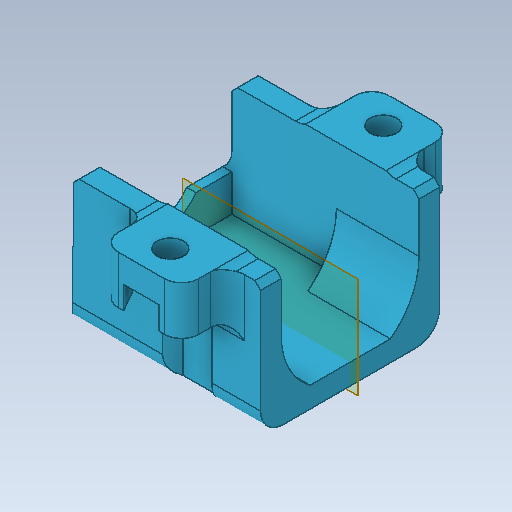
# Autodesk Inventor part: MotorTop
Saved by Autodesk Inventor 2025 (Build 290162000, 162)
## iProperties
Created: 2015-06-14
Part Number: MotorTop
Material: PC/ABS Plastic
Document SubType Name: Modeling
Designer: Lincoln
Density: 0.357273 g/cm^3
Appearance: Turquoise
Mass: 0.194626 g
Surface Area: 10.2421 cm^2
Volume: 0.544755 cm^3
Author: Lincoln
Autodesk Inventor part; units mm, degrees
ref_plane "YZ Plane" through (0, 0, 0) normal (1, 0, 0) x (0, 1, 0)
ref_plane "XZ Plane" through (0, 0, 0) normal (0, 1, 0) x (-1, 0, 0)
ref_plane "XY Plane" through (0, 0, 0) normal (0, 0, 1) x (1, 0, 0)
sketch "Sketch1" plane through (0, 0, 0) normal (1, 0, 0) x (0, 1, 0)
  line L0 (4.975, -6) -> (0, -6) construction
  line L1 (0, -6) -> (0, 0) construction
  line L2 (0, 0) -> (8.45, 0) construction
  line L3 (4.975, 6) -> (0, 6) construction
  line L4 (0, 6) -> (0, 0) construction
  line L5 (0, 6) -> (0, 7.8) construction
  line L6 (0, 7.8) -> (9.8, 7.8)
  line L7 (9.8, 7.8) -> (9.8, 6)
  line L8 (9.8, 6) -> (4.975, 6)
  line L9 (9.8, -6) -> (9.8, -7.8)
  line L10 (9.8, -7.8) -> (0, -7.8)
  line L11 (0, -7.8) -> (0, -6) construction
  line L12 (9.8, -6) -> (4.975, -6)
  line L13 (0, 7.8) -> (-1.8, 7.8)
  line L14 (-1.8, 7.8) -> (-1.8, -7.8)
  line L15 (-1.8, -7.8) -> (0, -7.8)
  circle A0 centre (4.975, -0.2001) radius 2.5 projected
  line L16 (9.95, -3.5) -> (9.95, 3.5) projected
  arc A1 (9.95, 3.5) -> (0, 3.5) centre (4.975, -0.2001) ccw projected
  line L17 (0, 3.5) -> (0, -3.5) projected
  arc A2 (0, -3.5) -> (9.95, -3.5) centre (4.975, 0.2001) ccw projected
  point P0 (0, 0)
  point P1 (4.975, 6)
  dimension "d8" = 0
  dimension "d22" = 1.8
  dimension "d23" = 9.8
  dimension "d24" = 1.8
  dimension "d25" = 1.8
  constraints: 32 end point, 7 perpendicular, 4 horizontal, 3 vertical, 1 collinear, 1 point on circle, 1 tangent, 4 other
  measures "d8" distance of L1.end point (0, 0)
  measures "d22" distance of L3.end L5.end
  measures "d23" distance of L5.end L6.end
  measures "d24" distance of L6.end L7.end
  measures "d25" distance of L5.end L13.end
extrude "Extrusion1" add sketch "Sketch1" along normal blind 15.2 contours L6 L7 L8 A1 L17 A2 L12 L9 L10 L15 L14 L13
sketch "Sketch2" plane through (0, -1.8, -7.8) normal (0, -1, 0) x (1, 0, 0)
  line L0 (-9.1, 0) -> (-9.1, 10.8)
  line L1 (-9.1, 10.8) -> (-9.1, 15.6)
  line L2 (-9.1, 15.6) -> (-9.9, 15.6)
  line L3 (-9.9, 15.6) -> (-9.9, 0)
  line L4 (-9.9, 0) -> (-9.1, 0)
  line L5 (0, 15.6) -> (15.2, 15.6) projected
  line L6 (0, 0) -> (15.2, 0) projected
  line L7 (0, 15.6) -> (0, 0) projected
  dimension "d30" = 0.8
  dimension "d141" = 9.1
  constraints: 10 end point, 3 perpendicular, 2 collinear, 1 point on line
  measures "d30" distance of L1.end L2.end
  measures "d141" distance between parallel lines of L7 L0
extrude "Extrusion2" add sketch "Sketch2" against normal blind 5
sketch "Sketch3" plane through (-9.1, -1.8, 7.8) normal (1, 0, 0) x (0, 0, -1)
  line L0 (0, 11.6) -> (0, 0) projected
  line L1 (0, 0) -> (15.6, 0) projected
  circle A0 centre (8.0001, 6.775) radius 2 projected
  arc A1 (13.8, 11.25) -> (13.3, 11.75) centre (13.3, 11.25) ccw projected
  line L2 (13.8, 11.25) -> (13.8, 2.3) projected
  arc A2 (13.3, 1.8) -> (13.8, 2.3) centre (13.3, 2.3) ccw projected
  line L3 (13.3, 1.8) -> (2.3, 1.8) projected
  arc A3 (1.8, 2.3) -> (2.3, 1.8) centre (2.3, 2.3) ccw projected
  line L4 (1.8, 2.3) -> (1.8, 11.25) projected
  arc A4 (2.3, 11.75) -> (1.8, 11.25) centre (2.3, 11.25) ccw projected
  line L5 (2.3, 11.75) -> (13.3, 11.75) projected
  line L6 (0, 11.6) -> (0, 0) projected
  line L7 (1.8, 11.6) -> (0, 11.6) projected
  line L8 (1.8, 6.775) -> (1.8, 11.6) projected
  arc A5 (1.8, 6.775) -> (4.3, 1.8) centre (8.0001, 6.775) ccw projected
  line L9 (11.3, 1.8) -> (4.3, 1.8) projected
  arc A6 (11.3, 1.8) -> (13.8, 6.775) centre (7.5999, 6.775) ccw projected
  line L10 (13.8, 11.6) -> (13.8, 6.775) projected
  line L11 (15.6, 11.6) -> (13.8, 11.6) projected
  line L12 (15.6, 0) -> (15.6, 11.6) projected
  line L13 (0, 0) -> (15.6, 0) projected
  point P0 (7.8, 1.8)
  point P1 (1.8, 9.8)
  point P2 (13.8, 9.8)
  point P3 (0, 1)
  point P4 (4.3, 1.8)
  point P5 (13.8, 6.775)
  point P6 (11.3, 1.8)
  point P7 (1.8, 6.775)
extrude "Extrusion3" add sketch "Sketch3" along normal blind 9.5 contours L7 L8 L4 A3 L3 A2 L2 L10 L11 L12 L1 L0 | A5 L3 A3 L4 | A6 L2 A2 L3
sketch "Sketch4" plane through (0, 0, 0) normal (-1, 0, 0) x (0, 0, 1)
  line L0 (-7.8, -1.8) -> (-7.8, 9.8) projected
  line L1 (-7.8, -1.8) -> (-7.8, 3.2) projected
  line L2 (-7.8, 3.2) -> (-7.8, 9.8) projected
  line L3 (7.8, 9.8) -> (7.8, -1.8) projected
  line L4 (7.8, 9.8) -> (7.8, 3.2) projected
  line L5 (7.8, -1.8) -> (7.8, 3.2) projected
  line L6 (7.8, -1.8) -> (-7.8, -1.8) projected
  line L7 (7.8, -1.8) -> (-7.8, -1.8) projected
  line L8 (-6, 9.8) -> (-6, 4.975) projected
  line L9 (-6, 9.8) -> (-6, 4.975) projected
  line L10 (6, 4.975) -> (6, 9.8) projected
  line L11 (6, 4.975) -> (6, 9.8) projected
  line L12 (-3.5, 0) -> (3.5, 0) projected
  line L13 (3.5, 0) -> (-3.5, 0) projected
  line L14 (-6, 4.975) -> (-6, 0)
  line L15 (-6, 0) -> (-3.5, 0)
  line L16 (6, 4.975) -> (6, 0)
  arc A0 (3.5, 0) -> (5.7405, 3.2) centre (-0.2001, 4.975) ccw projected
  line L17 (6, 0) -> (3.5, 0)
  line L18 (-7.8, 9.8) -> (-6, 9.8) projected
  line L19 (-7.8, 9.8) -> (-6, 9.8) projected
  line L20 (6, 9.8) -> (7.8, 9.8) projected
  line L21 (6, 9.8) -> (7.8, 9.8) projected
  arc A1 (-6, 4.975) -> (-3.5, 0) centre (0.2001, 4.975) ccw projected
  arc A2 (-6, 4.975) -> (-5.7405, 3.2) centre (0.2001, 4.975) ccw projected
  arc A3 (-5.7405, 3.2) -> (-3.5, 0) centre (0.2001, 4.975) ccw projected
  arc A4 (3.5, 0) -> (6, 4.975) centre (-0.2001, 4.975) ccw projected
  arc A5 (3.5, 0) -> (5.7405, 3.2) centre (-0.2001, 4.975) ccw projected
  arc A6 (5.7405, 3.2) -> (6, 4.975) centre (-0.2001, 4.975) ccw projected
  point P0 (0, 0)
  point P1 (-3.5, 0)
  point P2 (-6, 4.975)
  point P3 (-7.8, -1.8)
  point P4 (7.8, -1.8)
  point P5 (-3.5, 0)
  point P6 (-6, 4.975)
  constraints: 8 end point, 2 point on line, 1 horizontal, 1 perpendicular, 1 vertical
extrude "Extrusion4" cut sketch "Sketch4" along normal blind 9.1 contours A1 L15 L14 | L16 L17 A0 A4
sketch "Sketch5" plane through (15.2, 9.8, -7.8) normal (0, 0, -1) x (-1, 0, 0)
  line L0 (15.2, 0) -> (11.2, 0) construction
  line L1 (24.3, 0) -> (0, 0) construction
  line L2 (0, -11.6) -> (0, 0)
  line L3 (0, 0) -> (0, 0)
  line L4 (0, 0) -> (0, -6)
  line L5 (0, 0) -> (11.2, 0)
  line L6 (8, -11.6) -> (0, -11.6)
  line L7 (0, -11.6) -> (0, 0)
  line L8 (0, 0) -> (8, 0)
  line L9 (8, 0) -> (8, -11.6)
  line L10 (25.1, -11.6) -> (0, -11.6) projected
  dimension "d48" = 0
  dimension "d113" = 8
  constraints: 18 end point, 2 collinear, 2 parallel, 2 point on line, 1 horizontal, 1 perpendicular
  measures "d48" distance of L1.end L3.end
  measures "d113" distance between parallel lines of L2 L9
extrude "Extrusion5" cut sketch "Sketch5" against normal through all
sketch "Sketch10" plane through (0, 9.8, 7.2) normal (0, 1, 0) x (1, 0, 0)
  line L0 (-2.6843, -4.6) -> (4.3157, -4.6)
  line L1 (4.3157, -4.6) -> (4.3157, 0)
  line L2 (4.3157, 0) -> (-2.6843, 0) construction
  line L3 (-2.6843, 1.2) -> (-2.6843, -4.6)
  line L4 (0.8157, -4.6) -> (0.8157, 0) construction
  line L5 (-6.65, -2.0756) -> (1.3238, -2.0756) construction
  circle A0 centre (0.8157, -2.0756) radius 1.15
  line L6 (-5.9343, -1) -> (-5.9343, 11.4) construction
  line L7 (0, 1.2) -> (-2.6843, 1.2)
  line L8 (-9.1, 1.2) -> (7.2, 1.2) projected
  line L9 (-9.1, -0.6) -> (15.2, -0.6) projected
  circle A1 centre (0.8157, -2.0756) radius 1.1 projected
  line L10 (4.3157, 0) -> (4.3157, 1.2)
  line L11 (0, 1.2) -> (4.3157, 1.2)
  point P0 (0, 6.2)
  point P1 (0, -0.6)
  point P2 (7.2, -0.6)
  point P3 (-9.1, 0)
  point P4 (15.2, -0.6)
  dimension "d94" = 7
  dimension "d96" = 2.3
  dimension "d97" = 3.25
  dimension "d136" = 5.8
  constraints: 20 end point, 5 point on line, 3 horizontal, 3 perpendicular, 2 midpoint, 2 parallel, 1 centre point, 1 coincident, 2 other
  measures "d94" distance of L0.start L0.end
  measures "d96" diameter of A0
  measures "d97" distance between parallel lines of L3 L6
  measures "d136" distance of L3.start L0.start
extrude "Screw Hole" add sketch "Sketch10" along normal blind 0.2 and the other way blind 4 contours L3 L9 L1 L0 | L3 L7 L8 L10 L1 L9
sketch "Sketch11" plane through (0, 5.8, 7.2) normal (0, -1, 0) x (1, 0, 0)
  circle A0 centre (0.8157, 2.0756) radius 1.15 projected
  line L0 (-0.6843, 4.6737) -> (2.3157, 4.6737)
  line L1 (2.3157, 4.6737) -> (3.8157, 2.0756)
  line L2 (3.8157, 2.0756) -> (2.3157, -0.5224)
  line L3 (2.3157, -0.5224) -> (-0.6843, -0.5224)
  line L4 (-0.6843, -0.5224) -> (-2.1843, 2.0756)
  line L5 (-2.1843, 2.0756) -> (-0.6843, 4.6737)
  point P0 (0, -7.2)
  point P1 (-3.15, 0)
  point P2 (0.8157, 2.0756)
  dimension "d132" = 3
  constraints: 12 end point, 1 coincident, 1 horizontal, 14 other
  measures "d132" distance of L0.start L0.end
extrude "Extrusion10" cut sketch "Sketch11" along normal blind 10 and the other way blind 2
mirror "Mirror1" about plane through (0, 0, 0) normal (0, 0, 1) of "Screw Hole", "Extrusion10"
fillet "Fillet3" radius 1.5 2 edges at (-2.6843, 7.8, -7.8) (4.3157, 7.8, -7.8)
fillet "Fillet4" radius 1.5 1 edges at (4.3157, 7.9, 11.8)
fillet "Fillet5" radius 1.5 1 edges at (-2.6843, 7.9, 11.8)
fillet "Fillet6" radius 1.5 2 edges at (4.3157, 7.9, -11.8) (-2.6843, 7.9, -11.8)
fillet "Fillet7" radius 1.5 1 edges at (4.3157, 7.8, 7.8)
fillet "Fillet8" radius 1.5 1 edges at (-2.6843, 7.8, 7.8)
chamfer "Chamfer1" distance 0.7 angle 45 2 edges at (-9.9, 0.7, -7.8) (-9.9, 0.7, 7.8)
ref_plane "Work Plane2" through (7.2, -1.8, 0) normal (0, 0, -1) x (-1, 0, 0)
fillet "Fillet10" radius 2 2 edges at (5.0819, -1.8, 7.8) (5.0819, -1.8, -7.8)
fillet "Fillet11" radius 2 8 edges at (4.3157, 9.8, 8.55) (4.3157, 9.8, 6.9) (4.3157, 9.8, -8.55) (4.3157, 9.8, -6.9) (-2.6843, 9.8, -8.55) (-2.6843, 9.8, -6.9) (-2.6843, 9.8, 8.55) (-2.6843, 9.8, 6.9)
sketch "Sketch12" plane through (-9.9, 3.2, -7.1) normal (-1, 0, 0) x (0, 0, 1)
  circle A0 centre (6.8999, 1.775) radius 2.5 projected
  circle A1 centre (6.8999, 1.775) radius 3.2
  point P0 (7.1, -3.2)
  dimension "d144" = 6.4
  constraints: 1 centre point, 1 coincident
  measures "d144" diameter of A1
extrude "Extrusion11" cut sketch "Sketch12" against normal blind 1.8 contours A0 | A1
chamfer "Chamfer2" distance 0.5 angle 45 4 edges at (-9.1, 9.8, -6.9) (-9.1, 9.8, 6.9) (7.2, 9.8, 6.9) (7.2, 9.8, -6.9)
fillet "Fillet12" radius 2 2 edges at (-9.1, 3.2, 6.9) (-9.1, 3.2, -6.9)
fillet "Fillet13" radius 1 4 edges at (-2.7583, 5.8, 7.8) (4.3898, 5.8, 7.8) (4.3898, 5.8, -7.8) (-2.7583, 5.8, -7.8)
body "Solid1"
